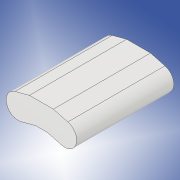
# Autodesk Inventor part: CA003
Saved by Autodesk Inventor 2017 (Build 210142000, 142)
## iProperties
Created: 2017-07-18
Part Number: CA003
Material: ABS Plastic
Document SubType Name: Modeling
Designer: zallen
Density: 1.06 g/cm^3
Appearance: CR White
Author: zallen
Autodesk Inventor part; units mm, degrees
ref_plane "YZ Plane" through (0, 0, 0) normal (1, 0, 0) x (0, 1, 0)
ref_plane "XZ Plane" through (0, 0, 0) normal (0, 1, 0) x (-1, 0, 0)
ref_plane "XY Plane" through (0, 0, 0) normal (0, 0, 1) x (1, 0, 0)
sketch "Sketch1" plane through (0, 0, 0) normal (0, 0, 1) x (1, 0, 0)
  line L0 (0, 0) -> (160, 0)
  line L1 (160, 0) -> (118.589, -154.5481)
  line L2 (0, 0) -> (41.411, -154.5481)
  line L3 (41.411, -154.5481) -> (118.589, -154.5481)
  dimension "d4" = 160
  dimension "d5" = 160
  dimension "d6" = 160
  dimension "d7" = 75
  constraints: 8 end point, 2 horizontal
  measures "d4" distance of L0.start L0.end
  measures "d5" distance of L0.end L1.end
  measures "d6" distance of L0.start L2.end
  measures "d7" angle of L0 L2
extrude "Extrusion1" add sketch "Sketch1" along normal blind 650
sketch "Sketch2" plane through (0, 0, 650) normal (0, 0, 1) x (1, 0, 0)
  circle A0 centre (235.8871, -103.156) radius 80 construction
  circle A1 centre (-75.8871, -103.156) radius 80 construction
  line L0 (160, 0) -> (0, 0) projected
  line L1 (-96.5926, -25.8819) -> (0, 0)
  line L2 (0, 0) -> (41.411, -154.5481) projected
  line L3 (-55.1815, -180.43) -> (41.411, -154.5481)
  line L4 (0, 0) -> (41.411, -154.5481)
  arc A2 (-96.5926, -25.8819) -> (-55.1815, -180.43) centre (-75.8871, -103.156) ccw
  line L5 (41.411, -154.5481) -> (118.589, -154.5481) projected
  line L6 (118.589, -154.5481) -> (215.1815, -180.43)
  line L7 (160, 0) -> (256.5926, -25.8819)
  arc A3 (215.1815, -180.43) -> (256.5926, -25.8819) centre (235.8871, -103.156) ccw
  line L8 (160, 0) -> (118.589, -154.5481)
  dimension "d8" = 160
  dimension "d9" = 160
  dimension "d10" = 100
  dimension "d13" = 100
  constraints: 12 end point, 8 point on circle, 7 tangent, 4 centre point, 1 parallel, 1 perpendicular
  measures "d8" diameter of A0
  measures "d9" diameter of A1
  measures "d10" distance of L1.start L0.end
  measures "d13" distance of L0.start L7.end
extrude "Extrusion2" add sketch "Sketch2" against normal blind 650 contours L7 A3 L6 L8 | L2 L3 A2 L1
body "Solid1"
